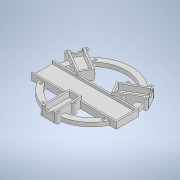
# Autodesk Inventor part: bottom2_turnigy
Saved by Autodesk Inventor 2020.4 (Build 244396000, 396)
## iProperties
Created: 2020-03-22
Part Number: bottom2_turnigy
Material: Generic
Document SubType Name: Modeling
Designer: Tarsoly
Density: 1 g/cm^3
Appearance: Default
Author: Tarsoly
Autodesk Inventor part; units mm, degrees
ref_plane "YZ Plane" through (0, 0, 0) normal (1, 0, 0) x (0, 1, 0)
ref_plane "XZ Plane" through (0, 0, 0) normal (0, 1, 0) x (-1, 0, 0)
ref_plane "XY Plane" through (0, 0, 0) normal (0, 0, 1) x (1, 0, 0)
sketch "Sketch1" plane through (0, 0, 0) normal (0, 1, 0) x (-1, 0, 0)
  circle A0 centre (0, 0) radius 50
  circle A1 centre (0, 0) radius 43
  line L0 (0, -70.9238) -> (0, 75.5426) construction
  line L1 (71.8218, 0) -> (-71.8218, 0) construction
  circle A2 centre (0, 0) radius 46.5 construction
  circle A3 centre (30.6145, -35) radius 1.5
  circle A4 centre (-30.6145, -35) radius 1.5
  circle A5 centre (-39.2078, 25) radius 1.5
  circle A6 centre (39.2078, 25) radius 1.5
  circle A7 centre (0, 0) radius 20.6188 construction
  line L2 (6, 22.6188) -> (-6, 22.6188) construction
  line L3 (-6, 22.6188) -> (-6, 52.6188) construction
  line L4 (-6, 52.6188) -> (6, 52.6188) construction
  line L5 (6, 52.6188) -> (6, 22.6188) construction
  line L6 (0, 22.6188) -> (0, 52.6188) construction
  line L7 (-8, 54.6188) -> (-8, 20.6188)
  line L8 (-8, 20.6188) -> (8, 20.6188)
  line L9 (8, 20.6188) -> (8, 54.6188)
  line L10 (8, 54.6188) -> (-8, 54.6188)
  line L11 (-48.5692, -21.1132) -> (-22.5885, -6.1132) construction
  line L12 (-16.5885, -16.5056) -> (-42.5692, -31.5056) construction
  line L13 (-43.3013, -34.2376) -> (-13.8564, -17.2376)
  line L14 (-51.3013, -20.3812) -> (-43.3013, -34.2376)
  line L15 (-42.5692, -31.5056) -> (-48.5692, -21.1132) construction
  line L16 (-21.8564, -3.3812) -> (-51.3013, -20.3812)
  line L17 (-13.8564, -17.2376) -> (-21.8564, -3.3812)
  line L18 (-22.5885, -6.1132) -> (-16.5885, -16.5056) construction
  line L19 (42.5692, -31.5056) -> (16.5885, -16.5056) construction
  line L20 (22.5885, -6.1132) -> (48.5692, -21.1132) construction
  line L21 (51.3013, -20.3812) -> (21.8564, -3.3812)
  line L22 (43.3013, -34.2376) -> (51.3013, -20.3812)
  line L23 (48.5692, -21.1132) -> (42.5692, -31.5056) construction
  line L24 (13.8564, -17.2376) -> (43.3013, -34.2376)
  line L25 (21.8564, -3.3812) -> (13.8564, -17.2376)
  line L26 (16.5885, -16.5056) -> (22.5885, -6.1132) construction
  point P0 (-45.5692, -26.3094)
  point P1 (-19.5885, -11.3094)
  point P2 (45.5692, -26.3094)
  point P3 (19.5885, -11.3094)
  point P4 (-8, 49.3559)
  point P5 (8, 49.3559)
  point P6 (8, 42.2493)
  point P7 (-8, 42.2493)
  point P8 (-40.5889, -14.1964)
  point P9 (-32.5889, -28.0528)
  point P10 (-38.7434, -31.6061)
  point P11 (-46.7434, -17.7497)
  point P12 (46.7434, -17.7497)
  point P13 (38.7434, -31.6061)
  point P14 (32.5889, -28.0528)
  point P15 (40.5889, -14.1964)
  dimension "d0" = 100
  dimension "d1" = 86
  dimension "d61" = 93
  dimension "d62" = 3
  dimension "d63" = 3
  dimension "d64" = 3
  dimension "d65" = 3
  dimension "d66" = 35
  dimension "d67" = 35
  dimension "d68" = 25
  dimension "d69" = 25
  dimension "d147" = 12
  dimension "d148" = 30
  dimension "d149" = 2
  dimension "d152" = 360
  dimension "d154" = 24
  constraints: 50 end point, 8 centre point, 4 coincident, 4 parallel, 4 point on circle, 2 midpoint, 2 perpendicular, 1 collinear, 1 horizontal, 1 tangent, 58 other
  measures "d0" diameter of A0
  measures "d1" diameter of A1
  measures "d61" diameter of A2
  measures "d62" diameter of A3
  measures "d63" diameter of A4
  measures "d64" diameter of A5
  measures "d65" diameter of A6
  measures "d66" distance from line of L1 A3.centre
  measures "d67" distance from line of L1 A4.centre
  measures "d68" distance from line of L1 A5.centre
  measures "d69" distance from line of L1 A6.centre
  measures "d147" distance of L3.end L4.end
  measures "d148" distance of L2.end L3.end
  measures "d149" distance between parallel lines of L3 L7
  measures "d154" distance from line of L8 L16.start
extrude "Extrusion1" add sketch "Sketch1" along normal blind 5 contours A0 L21 A1 L9 | L9 A1 L7 A0 | A0 L7 L10 L9 | L21 L22 L24 A0 | A0 L24 A1 L21 | L7 A1 L16 A0 | L9 L8 L7 A1 | A0 L13 A1 L24 | A1 L24 L25 L21 | L16 A1 L13 A0 | A0 L13 L14 L16 | L16 L17 L13 A1
sketch "Sketch6" plane through (0, 5, 0) normal (0, 1, 0) x (1, 0, 0)
  line L0 (-8, -20.6188) -> (-8, -42.2493) projected
  line L1 (8, -54.6188) -> (8, -49.3559) projected
  line L2 (-8, -20.6188) -> (8, -20.6188)
  line L3 (8, -20.6188) -> (8, -54.6188)
  line L4 (8, -54.6188) -> (-8, -54.6188)
  line L5 (-8, -54.6188) -> (-8, -20.6188)
  line L6 (6, -52.6188) -> (6, -22.6188)
  line L7 (6, -22.6188) -> (-6, -22.6188)
  line L8 (-6, -22.6188) -> (-6, -52.6188)
  line L9 (-6, -52.6188) -> (6, -52.6188)
  point P0 (0, 0)
  dimension "d156" = 2
  constraints: 16 end point, 4 parallel, 2 perpendicular, 1 horizontal, 3 other
  measures "d156" distance between parallel lines of L3 L6
extrude "Extrusion5" add sketch "Sketch6" along normal blind 7
sketch "Sketch7" plane through (-7, 0, 54.6188) normal (0, 0, 1) x (1, 0, 0)
  circle A0 centre (7, 10) radius 2.5
  line L0 (2.5, 10) -> (7, 10) construction
  line L1 (7, 10) -> (11.5, 10) construction
  circle A1 centre (2.5, 10) radius 1
  circle A2 centre (11.5, 10) radius 1
  line L2 (2.5, 11) -> (4.7087, 11)
  line L3 (2.5, 9) -> (4.7087, 9)
  line L4 (9.2913, 11) -> (11.5, 11)
  line L5 (9.2913, 9) -> (11.5, 9)
  line L6 (1.5, 12) -> (1.5, 10)
  line L7 (12.5, 12) -> (12.5, 10)
  line L8 (-1, 12) -> (15, 12) projected
  line L9 (1, 5) -> (13, 5) construction
  line L10 (-25.5889, 5) -> (39.5889, 5) construction
  line L11 (7, 5) -> (7, 10) construction
  point P0 (60.8748, 5)
  point P1 (-39.7434, 5)
  point P2 (53.7434, 5)
  dimension "d51" = 5
  dimension "d53" = 9
  dimension "d54" = 2
  dimension "d55" = 2
  dimension "d159" = 5
  constraints: 18 end point, 10 point on circle, 6 tangent, 4 horizontal, 3 centre point, 3 point on line, 2 coincident, 2 parallel, 2 perpendicular, 1 collinear, 1 midpoint
  measures "d51" diameter of A0
  measures "d53" distance of L1.end L0.start
  measures "d54" diameter of A1
  measures "d55" diameter of A2
  measures "d159" distance of L11.start L0.end
extrude "Extrusion14" cut sketch "Sketch7" against normal up to surface (2 mm away) contours A0 L8 | A0 L4 A2 L5 | A0 L8 L7 A2 L4 | A2 | L3 A1 L2 A0 | A0 L2 A1 L6 L8 | A1 picked at (6.1502, 9.8567)
sketch "Sketch16" plane through (0, 0, 0) normal (0, -1, 0) x (1, 0, 0)
  line L0 (8, 42.2493) -> (8, 20.6188) projected
  line L1 (8, 20.6188) -> (-8, 20.6188) projected
  line L2 (-8, 20.6188) -> (-8, 42.2493) projected
  line L3 (-8, 49.3559) -> (-8, 54.6188) construction
  line L4 (-8, 54.6188) -> (8, 54.6188) projected
  line L5 (8, 54.6188) -> (8, 49.3559) projected
  line L6 (-20.9087, 28.8188) -> (39.4315, 28.8188) construction
  circle A0 centre (-9, 52.1188) radius 1
  circle A1 centre (-9, 52.1188) radius 2.5
  line L7 (-8, 20.6188) -> (-8, 54.6188) projected
  line L8 (-8, 54.6188) -> (8, 54.6188) projected
  circle A2 centre (9, 52.1188) radius 1
  circle A3 centre (9, 52.1188) radius 2.5
  circle A4 centre (-9, 31.1188) radius 1
  circle A5 centre (-9, 31.1188) radius 2.5
  circle A6 centre (9, 31.1188) radius 1
  circle A7 centre (9, 31.1188) radius 2.5
  point P0 (0, 0)
  point P1 (-5.5, 54.6188)
  point P2 (-8, 33.4101)
  point P3 (-8, 28.8275)
  point P4 (-8, 31.1188)
  point P5 (-8, 52.1188)
  point P6 (-8, 54.4101)
  point P7 (-8, 49.8275)
  point P8 (8, 54.4101)
  point P9 (8, 52.1188)
  point P10 (8, 49.8275)
  point P11 (8, 33.4101)
  point P12 (8, 31.1188)
  point P13 (8, 28.8275)
  dimension "d162" = 25.8
  dimension "d163" = 2
  dimension "d164" = 1.5
  dimension "d165" = 16
  dimension "d168" = 18
  dimension "d171" = 21
  constraints: 8 centre point, 2 end point, 2 horizontal, 2 tangent, 1 vertical, 9 other
  measures "d162" distance between parallel lines of L4 L6
  measures "d163" diameter of A0
  measures "d164" radial gap between concentric circles of A0 A1
  measures "d165" distance of L0.end L1.end
  measures "d168" distance of A0.centre A2.centre
  measures "d171" distance of A0.centre A4.centre
extrude "Extrusion15" add sketch "Sketch16" against normal up to surface (12 mm away) contours A7 L0 | A5 L2 | A3 L5 | L5 A3 | L7 A1 picked at (10.9649, 30.8346) picked at (-10.9649, 30.8346) picked at (-10.9649, 51.8346)
pattern_circular "Circular Pattern3" count 3 over 360 about axis through (0, -10, 0) along (0, 1, 0) of "Extrusion5", "Extrusion14", "Extrusion15"
sketch "Sketch11" plane through (0, 0, 0) normal (0, -1, 0) x (1, 0, 0)
  arc A0 (-8, 42.2493) -> (-40.5889, -14.1964) centre (0, 0) ccw projected
  circle A1 centre (39.2078, 25) radius 1.5 projected
  circle A2 centre (-39.2078, 25) radius 1.5 projected
  circle A3 centre (30.6145, -35) radius 1.5 projected
  circle A4 centre (-30.6145, -35) radius 1.5 projected
  line L0 (8, 54.6188) -> (8, 54.4101) projected
  line L1 (-8, 54.6188) -> (8, 54.6188) projected
  line L2 (-8, 49.3559) -> (-8, 49.8275) projected
  arc A5 (-8, 49.3559) -> (-46.7434, -17.7497) centre (0, 0) ccw projected
  line L3 (-51.3013, -20.3812) -> (-51.1205, -20.2768) projected
  line L4 (-43.3013, -34.2376) -> (-51.3013, -20.3812) projected
  line L5 (-38.7434, -31.6061) -> (-39.1519, -31.842) projected
  arc A6 (-38.7434, -31.6061) -> (38.7434, -31.6061) centre (0, 0) ccw projected
  line L6 (43.3013, -34.2376) -> (43.1205, -34.1332) projected
  line L7 (51.3013, -20.3812) -> (43.3013, -34.2376) projected
  line L8 (46.7434, -17.7497) -> (47.1519, -17.9856) projected
  line L9 (-8, 20.6188) -> (-8, 28.8275) projected
  line L10 (8, 20.6188) -> (-8, 20.6188) projected
  line L11 (8, 42.2493) -> (8, 33.4101) projected
  arc A7 (40.5889, -14.1964) -> (8, 42.2493) centre (0, 0) ccw projected
  line L12 (21.8564, -3.3812) -> (28.9654, -7.4856) projected
  line L13 (13.8564, -17.2376) -> (21.8564, -3.3812) projected
  line L14 (32.5889, -28.0528) -> (24.934, -23.6332) projected
  arc A8 (-32.5889, -28.0528) -> (32.5889, -28.0528) centre (0, 0) ccw projected
  line L15 (-13.8564, -17.2376) -> (-20.9654, -21.342) projected
  line L16 (-21.8564, -3.3812) -> (-13.8564, -17.2376) projected
  line L17 (-40.5889, -14.1964) -> (-32.934, -9.7768) projected
  arc A9 (39.1519, -31.842) -> (43.1205, -34.1332) centre (40.6362, -33.8536) ccw projected
  arc A10 (51.1205, -20.2768) -> (47.1519, -17.9856) centre (49.6362, -18.2652) ccw projected
  arc A11 (8, 49.8275) -> (8, 54.4101) centre (9, 52.1188) ccw projected
  arc A12 (-8, 54.4101) -> (-8, 49.8275) centre (-9, 52.1188) ccw projected
  arc A13 (46.7434, -17.7497) -> (8, 49.3559) centre (0, 0) ccw projected
  arc A14 (-47.1519, -17.9856) -> (-51.1205, -20.2768) centre (-49.6362, -18.2652) ccw projected
  arc A15 (-43.1205, -34.1332) -> (-39.1519, -31.842) centre (-40.6362, -33.8536) ccw projected
  line L18 (-8, 33.4101) -> (-8, 42.2493) projected
  arc A16 (-8, 33.4101) -> (-8, 28.8275) centre (-9, 31.1188) ccw projected
  line L19 (8, 28.8275) -> (8, 20.6188) projected
  arc A17 (8, 28.8275) -> (8, 33.4101) centre (9, 31.1188) ccw projected
  line L20 (32.934, -9.7768) -> (40.5889, -14.1964) projected
  arc A18 (32.934, -9.7768) -> (28.9654, -7.4856) centre (31.4497, -7.7652) ccw projected
  line L21 (20.9654, -21.342) -> (13.8564, -17.2376) projected
  arc A19 (20.9654, -21.342) -> (24.934, -23.6332) centre (22.4497, -23.3536) ccw projected
  line L22 (-24.934, -23.6332) -> (-32.5889, -28.0528) projected
  arc A20 (-24.934, -23.6332) -> (-20.9654, -21.342) centre (-22.4497, -23.3536) ccw projected
  line L23 (-28.9654, -7.4856) -> (-21.8564, -3.3812) projected
  arc A21 (-28.9654, -7.4856) -> (-32.934, -9.7768) centre (-31.4497, -7.7652) ccw projected
  circle A22 centre (-40.6362, -33.8536) radius 1 projected
  circle A23 centre (-9, 52.1188) radius 1 projected
  circle A24 centre (49.6362, -18.2652) radius 1 projected
  circle A25 centre (-49.6362, -18.2652) radius 1 projected
  circle A26 centre (9, 52.1188) radius 1 projected
  circle A27 centre (40.6362, -33.8536) radius 1 projected
  line L24 (39.1519, -31.842) -> (38.7434, -31.6061) projected
  line L25 (51.1205, -20.2768) -> (51.3013, -20.3812) projected
  line L26 (8, 49.8275) -> (8, 49.3559) projected
  line L27 (-8, 54.4101) -> (-8, 54.6188) projected
  line L28 (-47.1519, -17.9856) -> (-46.7434, -17.7497) projected
  line L29 (-43.1205, -34.1332) -> (-43.3013, -34.2376) projected
hole "Hole1" at (-39.2078, 0, 25) at (39.2078, 0, 25) at (30.6145, 0, -35) at (-30.6145, 0, -35) direction (0, 1, 0) diameter 3.2 depth 5 tip angle 118 clearance for "Hex Head Cap Screw ISO 24017" size "M3" standard "ISO"
sketch "Sketch17" plane through (0, 0, 0) normal (0, -1, 0) x (1, 0, 0)
  line L0 (-51.5, -3.3812) -> (51.5, -3.3812) construction
  line L1 (51.5, -3.3812) -> (51.5, 20.6188) construction
  line L2 (51.5, 20.6188) -> (-51.5, 20.6188) construction
  line L3 (-51.5, 20.6188) -> (-51.5, -3.3812) construction
  line L4 (8, 20.6188) -> (-8, 20.6188) construction
  line L5 (0, -3.3812) -> (0, 20.6188) construction
  line L6 (53.5, 22.6188) -> (53.5, -5.3812)
  line L7 (53.5, -5.3812) -> (-53.5, -5.3812)
  line L8 (-53.5, -5.3812) -> (-53.5, 22.6188)
  line L9 (-53.5, 22.6188) -> (53.5, 22.6188)
  line L10 (48.5, -0.3812) -> (-48.5, -0.3812)
  line L11 (-48.5, -0.3812) -> (-48.5, 17.6188)
  line L12 (-48.5, 17.6188) -> (48.5, 17.6188)
  line L13 (48.5, 17.6188) -> (48.5, -0.3812)
  arc A0 (-8, 49.3559) -> (-46.7434, -17.7497) centre (0, 0) ccw projected
  arc A1 (46.7434, -17.7497) -> (8, 49.3559) centre (0, 0) ccw projected
  arc A2 (-8, 49.3559) -> (-46.7434, -17.7497) centre (0, 0) ccw projected
  point P0 (48.5, 12.1552)
  point P1 (-48.5, 12.1552)
  point P2 (-46.7929, 17.6188)
  point P3 (46.7929, 17.6188)
  point P4 (47.769, -14.7688)
  point P5 (11.0943, 48.7536)
  point P6 (48.5, 12.1552)
  point P7 (46.7929, 17.6188)
  point P8 (-47.769, -14.7688)
  point P9 (-11.0943, 48.7536)
  point P10 (-48.5, 12.1552)
  point P11 (-46.7929, 17.6188)
  dimension "d176" = 103
  dimension "d177" = 24
  dimension "d178" = 2
  dimension "d179" = 3
  constraints: 26 end point, 6 parallel, 3 perpendicular, 2 midpoint, 1 collinear, 1 horizontal, 1 point on line, 6 other
  measures "d176" distance of L2.end L1.end
  measures "d177" distance of L1.end L0.end
  measures "d178" distance between parallel lines of L1 L6
  measures "d179" distance between parallel lines of L0 L10
extrude "Extrusion16" add sketch "Sketch17" against normal up to surface (5 mm away)
sketch "Sketch18" plane through (0, 5, 0) normal (0, 1, 0) x (1, 0, 0)
  line L0 (-53.5, -22.6188) -> (-53.5, 5.3812) projected
  line L1 (53.5, -22.6188) -> (44.5914, -22.6188) projected
  line L2 (-53.5, 5.3812) -> (53.5, 5.3812)
  line L3 (53.5, 5.3812) -> (53.5, -22.6188)
  line L4 (53.5, -22.6188) -> (-53.5, -22.6188)
  line L5 (-53.5, -22.6188) -> (-53.5, 5.3812)
  line L6 (51.5, -20.6188) -> (51.5, 3.3812)
  line L7 (51.5, 3.3812) -> (-51.5, 3.3812)
  line L8 (-51.5, 3.3812) -> (-51.5, -20.6188)
  line L9 (-51.5, -20.6188) -> (51.5, -20.6188)
  line L10 (-51.5, 3.3812) -> (-53.5, 3.3812)
  line L11 (-51.5, -20.6188) -> (-53.5, -20.6188)
  point P0 (0, 0)
  point P1 (-53.5, 3.3812)
  point P2 (-53.5, -20.6188)
  point P3 (-53.5, -22.6188)
  dimension "d182" = 2
  constraints: 20 end point, 4 parallel, 4 perpendicular, 2 point on line, 1 horizontal, 3 other
  measures "d182" distance between parallel lines of L3 L6
extrude "Extrusion17" add sketch "Sketch18" along normal blind 3 contours L0 L11 L9 L6 L7 L10 L2 L3 L1 L4
equation "\"d61\" = 0.5 * d1 + 0.5 * d0"
body "Solid1"
